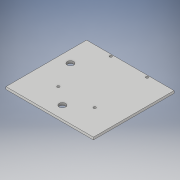
# Autodesk Inventor part: КВ33.044.002 - Дно платы
Saved by Autodesk Inventor 2019 (Build 230136000, 136)
## iProperties
Created: 2019-10-30
Part Number: КВ33.044.002 - Дно платы
Material: Типовые
Document SubType Name: Modeling
Designer: Петров Иван
Density: 1 g/cm^3
Appearance: По умолчанию
Author: Петров Иван
Autodesk Inventor part; units mm, degrees
ref_plane "YZ Plane" through (0, 0, 0) normal (1, 0, 0) x (0, 1, 0)
ref_plane "XZ Plane" through (0, 0, 0) normal (0, 1, 0) x (-1, 0, 0)
ref_plane "XY Plane" through (0, 0, 0) normal (0, 0, 1) x (1, 0, 0)
sketch "Эскиз1" plane through (0, 0, 0) normal (0, 1, 0) x (-1, 0, 0)
  line L0 (-25, 35) -> (25, 35)
  line L1 (25, 35) -> (25, -35)
  line L2 (25, -35) -> (-25, -35)
  line L3 (-25, -35) -> (-25, 35)
  line L4 (25, 35) -> (-25, -35) construction
  line L5 (-22.5, 32.5) -> (22.5, 32.5)
  line L6 (22.5, 31.5) -> (22.5, -31)
  line L7 (22.5, -32.5) -> (-22.5, -32.5)
  line L8 (-21.6462, 31.2667) -> (22.5, -32.5) construction
  line L9 (22.5, 32.5) -> (-22.5, -32.5) construction
  circle A0 centre (22.5, 32.5) radius 1.5
  circle A1 centre (22.5, -32.5) radius 1.5
  circle A2 centre (-22.5, -32.5) radius 1.5
  circle A3 centre (-22.5, 32.5) radius 1.5
  line L10 (-25, 35) -> (-23.7767, 33.2874) construction
  line L11 (-22.5, -31) -> (-22.5, 31)
  line L12 (-22.1692, 31.0369) -> (22.1692, -31.0369) construction
  line L13 (23.7767, -33.2874) -> (25, -35) construction
  line L14 (25, 35) -> (55, 35)
  line L15 (25, -30.9585) -> (25, 35)
  line L16 (25, 35) -> (-25, 35)
  line L17 (-25, 35) -> (-25, 65)
  line L18 (-25, 65) -> (25, 65)
  line L19 (25, 65) -> (25, 35)
  line L20 (55, 35) -> (25, 35)
  line L21 (25, 35) -> (25, 65)
  line L22 (25, 65) -> (55, 65)
  line L23 (55, 65) -> (55, 35)
  line L24 (0, 65) -> (0, 50)
  circle A4 centre (0, 50) radius 4
  line L25 (-25, 65) -> (-53.4747, 65)
  line L26 (-53.4747, 65) -> (-53.4747, -35)
  line L27 (-53.4747, -35) -> (-25, -35)
  line L28 (-25, -35) -> (-25, 65)
  line L29 (25, 35) -> (25, -35)
  line L30 (55, 35) -> (55, -35)
  line L31 (55, -35) -> (25, -35)
  line L32 (55, 0) -> (40, 0)
  circle A5 centre (40, 0) radius 4
  point P0 (0, 0)
  dimension "d6" = 3
  dimension "d0" = 50
  dimension "d2" = 45
  dimension "d4" = 3
  dimension "d5" = 3
  dimension "d7" = 3
  dimension "d9" = 30
  dimension "d11" = 15
  dimension "d12" = 8
  dimension "d16" = 15
  dimension "d17" = 8
  constraints: 66 end point, 10 parallel, 7 horizontal, 7 point on circle, 6 coincident, 5 centre point, 5 midpoint, 5 perpendicular, 4 point on line, 2 vertical, 1 collinear, 1 vertical alignment, 2 other
  measures "d0" distance of L1.end L2.end
  measures "d2" distance of L7.start L7.end
  measures "d4" diameter of A0
  measures "d5" diameter of A1
  measures "d7" diameter of A3
  measures "d9" distance of L16.end L17.end
  measures "d11" distance of L24.start L24.end
  measures "d12" diameter of A4
  measures "d16" distance of L32.start L32.end
  measures "d17" diameter of A5
extrude "Выдавливание1" add sketch "Эскиз1" along normal blind 3 contours L17 L18 L19 L0 | L0 L1 L2 L3 | L3 L27 L26 L25 L17 | L14 L30 L31 L1 | L19 L22 L23 L14 | L5 A0 L6 A1 L7 A2 L11 A3
